Autodesk Fusion 360 part; units mm, degrees
note: some values were not read from the file. Set by a fixed rule: which sketch regions a step uses.
(part 3 of 5)
extrude "Extrude3" cut sketch "Sketch3" against normal blind 0.5 contours L4 L24 L28 L40 L47 L50 L76 L81 L84 L116 L125 L129 L150 L155 L178 L210 L218 L225 L257 L304 L305 L332 L361 L386 L393 L479 L493 L497 L500 L526 L555 L557 L582 L587 L593 L598 L619 L670 L671 L694 L751 L783 L835 L871 L904 L934 L942 L946 L947 L982 L993 L997 L1046 L1064 L1093 L1098 L1104 L1114 L1123 L1124 L1129 L1137 L1150 L1158 L1165 L1171 L1172 L1176 L1181 L1189 L1191 L1213 L1217 L1219 L1221 L1234 L1256 L1262 L1266 L1284 L1287 L1293 L1300 L1301 L1641 L1649 | L5 L15 L17 L21 L38 L41 L43 L49 L59 L61 L88 L107 L123 L132 L157 L161 L208 L221 L227 L247 L256 L262 L264 L279 L300 L345 L359 L366 L367 L390 L394 L395 L403 L405 L423 L433 L494 L502 L515 L531 L534 L535 L548 L553 L576 L595 L655 L672 L678 L724 L733 L787 L806 L822 L852 L853 L861 L864 L870 L920 L961 L970 L976 L989 L995 L1000 L1001 L1004 L1015 L1018 L1027 L1039 L1068 L1069 L1099 L1105 L1140 L1143 L1161 L1168 L1175 L1195 L1196 L1210 L1224 L1240 L1269 L1377 L1625 | L6 L18 L26 L32 L44 L51 L55 L57 L70 L71 L72 L90 L91 L95 L99 L105 L106 L109 L113 L117 L118 L119 L126 L130 L137 L140 L143 L144 L146 L147 L169 L181 L185 L186 L188 L190 L206 L229 L232 L236 L240 L248 L253 L259 L260 L263 L269 L270 L286 L288 L291 L296 L301 L312 L323 L329 L330 L338 L341 L346 L358 L362 L372 L383 L384 L391 L392 L404 L417 L424 L445 L448 L451 L452 L453 L462 L476 L480 L482 L485 L498 L501 L513 L516 L523 L533 L536 L540 L543 L547 L558 L571 L573 L586 L589 L596 L607 L617 L623 L628 L631 L637 L656 L667 L669 L676 L697 L701 L703 L707 L715 L723 L727 L731 L732 L735 L736 L743 L744 L749 L755 L761 L774 L782 L790 L794 L800 L803 L805 L815 L823 L826 L828 L831 L839 L840 L850 L863 L866 L867 L872 L874 L875 L878 L883 L887 L894 L896 L902 L908 L912 L918 L933 L939 L945 L950 L957 L964 L966 L972 L978 L980 L984 L986 L987 L999 L1002 L1008 L1012 L1013 L1016 L1040 L1043 L1044 L1054 L1059 L1062 L1066 L1071 L1072 L1075 L1078 L1079 L1081 L1088 L1094 L1095 L1103 L1106 L1108 L1110 L1111 L1112 L1113 L1131 L1132 L1134 L1141 L1145 L1148 L1159 L1163 L1164 L1169 L1177 L1179 L1185 L1186 L1187 L1207 L1208 L1209 L1211 L1226 L1238 L1243 L1244 L1245 L1246 L1252 L1255 L1264 L1281 L1283 L1294 L1297 L1302 L1331 L1371 L1469 L1482 L1483 L1555 L1574 L1575 L1576 L1580 L1590 L1615 L1616 L1617 L1618 L1619 L1631 L1636 L1644 L1647 L1655 | L7 L8 L14 L25 L31 L33 L48 L100 L111 L134 L151 L164 L173 L183 L191 L197 L198 L200 L201 L209 L216 L223 L233 L246 L252 L258 L265 L278 L281 L282 L314 L324 L327 L335 L336 L339 L348 L364 L369 L382 L387 L388 L389 L407 L408 L411 L414 L415 L426 L435 L438 L441 L442 L446 L449 L456 L457 L458 L469 L470 L475 L477 L478 L484 L488 L492 L496 L504 L507 L510 L511 L512 L517 L519 L521 L524 L529 L532 L539 L542 L545 L546 L549 L550 L552 L559 L562 L567 L575 L577 L578 L580 L583 L592 L597 L600 L606 L608 L612 L613 L616 L618 L620 L624 L626 L629 L632 L633 L635 L639 L640 L641 L642 L643 L644 L646 L647 L649 L650 L653 L658 L659 L660 L661 L662 L663 L665 L668 L673 L674 L679 L681 L683 L684 L685 L686 L690 L691 L692 L693 L695 L696 L700 L702 L705 L710 L713 L726 L737 L739 L756 L758 L759 L763 L764 L765 L770 L780 L781 L785 L789 L791 L793 L795 L799 L801 L811 L813 L817 L821 L837 L842 L845 L847 L848 L851 L855 L857 L858 L859 L860 L877 L890 L891 L936 L937 L1041 L1120 L1147 L1149 L1180 L1183 L1199 L1203 L1206 L1257 L1304 L1306 L1307 L1308 L1309 L1310 L1312 L1313 L1314 L1315 L1317 L1319 L1320 L1321 L1322 L1323 L1325 L1326 L1327 L1328 L1332 L1333 L1334 L1335 L1336 L1337 L1339 L1342 L1367 L1368 L1369 L1372 L1373 L1374 L1375 L1376 L1379 L1380 L1389 L1390 L1391 L1392 L1393 L1394 L1395 L1396 L1398 L1399 L1400 L1401 L1406 L1410 L1411 L1412 L1414 L1415 L1418 L1450 L1452 L1453 L1454 L1455 L1456 L1457 L1458 L1459 L1460 L1461 L1462 L1463 L1464 L1465 L1466 L1467 L1468 | L9 L20 L35 L63 L73 L83 L85 L97 L101 L156 L162 L168 L176 L177 L193 L205 L212 L235 L239 L241 L294 L353 L397 L413 L455 L471 L503 L508 L544 L565 L572 L585 L664 L666 L677 L688 L718 L740 L767 L775 L788 L809 L819 L830 L854 L865 L886 L888 L909 L913 L935 L949 L979 L991 L992 L994 L996 L1038 L1047 L1049 L1067 L1080 L1096 L1117 L1128 L1138 L1142 L1144 L1152 L1153 L1155 L1166 L1174 L1201 L1204 L1205 L1235 L1239 L1241 L1277 L1318 L1620 L1621 L1622 L1623 L1624 L1626 L1627 L1628 L1629 | L10 L13 L58 L66 L75 L78 L79 L86 L98 L120 L142 L196 L204 L234 L261 L298 L373 L385 L422 L454 L474 L486 L528 L591 L615 L675 L680 L689 L719 L762 L818 L820 L825 L829 L879 L884 L885 L893 L907 L916 L928 L967 L983 L990 L1007 L1009 L1017 L1035 L1050 L1063 L1074 L1121 L1139 L1167 L1170 L1173 L1271 L1291 L1630 L1633 L1638 L1639 L1648 L1650 L1651 L1652 | L11 L22 L53 L62 L68 L82 L104 L133 L152 L172 L226 L242 L250 L360 L379 L412 L443 L489 L505 L509 L525 L561 L574 L601 L622 L636 L645 L711 L717 L722 L772 L802 L814 L849 L882 L900 L903 L906 L919 L932 L938 L963 L965 L1051 L1053 L1077 L1109 L1127 L1133 L1136 L1222 L1232 L1237 L1249 L1259 L1289 L1290 L1365 L1428 L1637 L1640 L1646 L1653 L1654 | L12 L19 L27 L29 L30 L36 L37 L42 L45 L46 L52 L54 L56 L60 L67 L69 L74 L77 L80 L87 L89 L93 L94 L102 L110 L112 L114 L115 L124 L131 L135 L136 L138 L141 L153 L159 L160 L167 L171 L175 L180 L192 L199 L202 L217 L220 L224 L228 L230 L231 L244 L245 L251 L266 L283 L287 L290 L297 L299 L303 L307 L309 L315 L321 L322 L328 L331 L333 L334 L349 L352 L354 L365 L368 L370 L376 L396 L398 L399 L402 L427 L450 L460 L465 L468 L472 L483 L487 L490 L491 L495 L514 L520 L522 L527 L537 L541 L551 L554 L560 L563 L566 L568 L570 L579 L584 L602 L604 L611 L651 L657 L682 L698 L704 L706 L708 L709 L720 L741 L747 L748 L750 L760 L768 L769 L773 L778 L808 L816 L824 L827 L832 L834 L846 L862 L868 L869 L876 L881 L889 L895 L910 L911 L914 L926 L927 L929 L944 L948 L951 L962 L971 L977 L981 L985 L988 L998 L1005 L1006 L1010 L1026 L1045 L1055 L1061 L1065 L1070 L1073 L1085 L1091 L1092 L1097 L1118 L1125 L1146 L1151 L1156 L1157 L1160 L1162 L1178 L1182 L1188 L1200 L1220 L1227 L1248 L1251 L1253 L1265 L1274 L1275 L1279 L1286 L1292 L1295 L1296 L1298 L1303 L1370 L1632 L1634 L1635 L1642 L1643 L1645 L1656 | L16 L23 L39 L64 L92 L108 L121 L122 L127 L128 L139 L145 L148 L149 L154 L158 L165 L166 L170 L187 L189 L194 L211 L219 L237 L255 L268 L271 L273 L275 L280 L292 L293 L306 L313 L316 L319 L337 L347 L356 L371 L421 L447 L461 L518 L569 L610 L621 L638 L648 L652 L687 L712 L716 L728 L779 L796 L804 L838 L841 L843 L873 L892 L898 L899 L901 L915 L917 L921 L922 L924 L925 L930 L931 L940 L941 L943 L954 L959 L968 L969 L973 L974 L1003 L1011 L1014 L1019 L1020 L1028 L1029 L1030 L1031 L1032 L1033 L1034 L1036 L1037 L1042 L1048 L1052 L1056 L1057 L1058 L1060 L1076 L1082 L1083 L1084 L1086 L1087 L1089 L1090 L1101 L1107 L1115 L1116 L1122 L1130 L1135 L1154 L1184 L1192 L1193 L1194 L1198 L1202 L1216 L1218 L1225 L1231 L1233 L1236 L1242 L1247 L1250 L1261 L1268 L1270 L1273 L1285 L1299 | L34 L163 L203 L207 L243 L254 L284 L289 L317 L363 L418 L420 L425 L444 L466 L473 L499 L506 L564 L588 L590 L594 L609 L654 L725 L771 L797 L880 L1230 L1278 L1305 L1311 L1316 L1324 L1329 L1330 L1338 L1340 L1341 L1343 L1344 L1345 L1346 L1347 L1348 L1349 L1350 L1351 L1352 L1353 L1354 L1355 L1356 L1357 L1358 L1359 L1360 L1361 L1362 L1363 L1364 L1366 L1378 L1381 L1382 L1383 L1384 L1385 L1386 L1387 L1388 L1397 L1402 L1403 L1404 L1405 L1407 L1408 L1409 L1413 L1416 L1417 L1419 L1420 L1421 L1422 L1423 L1424 L1425 L1426 L1427 L1429 L1430 L1431 L1432 L1433 L1434 L1435 L1436 L1437 L1438 L1439 L1440 L1441 L1442 L1443 L1444 L1445 L1446 L1447 L1448 L1449 L1451 L1470 L1471 L1472 L1473 L1474 L1475 L1476 L1477 L1478 L1479 L1480 L1481 L1484 L1485 L1486 L1487 L1488 L1489 L1490 L1491 L1492 L1493 L1494 L1495 L1496 L1497 L1498 L1499 L1500 L1501 L1502 L1503 L1504 L1505 L1506 L1507 L1508 L1509 L1510 L1511 L1512 L1513 L1514 L1515 L1516 L1517 L1518 L1519 L1520 L1521 L1522 L1523 L1524 L1525 L1526 L1527 L1528 L1529 L1530 L1531 L1532 L1533 L1534 L1535 L1536 L1537 L1538 L1539 L1540 L1541 L1542 L1543 L1544 L1545 L1546 L1547 L1548 L1549 L1550 L1551 L1552 L1553 L1554 L1556 L1557 L1558 L1559 L1560 L1561 L1562 L1563 L1564 L1565 L1566 L1567 L1568 L1569 L1570 L1571 L1572 L1573 L1577 L1578 L1579 L1581 L1582 L1583 L1584 L1585 L1586 L1587 L1588 L1589 L1591 L1592 L1593 L1594 L1595 L1596 L1597 L1598 L1599 L1600 L1601 L1602 L1603 L1604 L1605 L1606 L1607 L1608 L1609 L1610 L1611 L1612 L1613 L1614 | L65 L96 L103 L174 L179 L182 L184 L195 L213 L214 L215 L222 L238 L249 L267 L272 L274 L276 L277 L285 L295 L302 L308 L310 L311 L318 L320 L325 L326 L340 L342 L343 L344 L350 L351 L355 L357 L374 L375 L377 L378 L380 L381 L400 L401 L406 L409 L410 L416 L419 L428 L429 L430 L431 L432 L434 L436 L437 L439 L440 L459 L463 L464 L481 L530 L538 L556 L581 L599 L603 L605 L614 L625 L627 L630 L634 L699 L714 L721 L729 L730 L734 L738 L742 L745 L746 L752 L753 L754 L757 L766 L776 L777 L784 L786 L792 L798 L807 L810 L812 L833 L836 L844 L856 L897 L905 L923 L952 L953 L955 L956 L958 L960 L975 L1021 L1022 L1023 L1024 L1025 L1100 L1102 L1119 L1126 L1190 L1197 L1212 L1214 L1215 L1223 L1228 L1229 L1254 L1258 L1260 L1263 L1267 L1272 L1276 L1280 L1288 in component "PCB Cover"
sketch "DXF" plane through (0, 0, 3) normal (0, 0, 1) x (-1, 0, 0)
  line L0 (-47.0979, -80.9274) -> (-46.9857, -80.9562)
  line L1 (-46.9857, -80.9562) -> (-46.8782, -80.9955)
  line L2 (-46.8782, -80.9955) -> (-46.7759, -81.0448)
  line L3 (-46.7759, -81.0448) -> (-46.6794, -81.1034)
  line L4 (-46.6794, -81.1034) -> (-46.5893, -81.1708)
  line L5 (-46.5893, -81.1708) -> (-46.5062, -81.2463)
  line L6 (-46.5062, -81.2463) -> (-46.4306, -81.3294)
  line L7 (-46.4306, -81.3294) -> (-46.3632, -81.4195)
  line L8 (-46.3632, -81.4195) -> (-46.3046, -81.516)
  line L9 (-46.3046, -81.516) -> (-46.2553, -81.6183)
  line L10 (-46.2553, -81.6183) -> (-46.2159, -81.7259)
  line L11 (-46.2159, -81.7259) -> (-46.187, -81.8381)
  line L12 (-46.187, -81.8381) -> (-46.1692, -81.9544)
  line L13 (-46.1692, -81.9544) -> (-46.1632, -82.0741)
  line L14 (-46.1632, -82.0741) -> (-46.1692, -82.1938)
  line L15 (-46.1692, -82.1938) -> (-46.187, -82.31)
  line L16 (-46.187, -82.31) -> (-46.2159, -82.4222)
  line L17 (-46.2159, -82.4222) -> (-46.2553, -82.5297)
  line L18 (-46.2553, -82.5297) -> (-46.3046, -82.632)
  line L19 (-46.3046, -82.632) -> (-46.3632, -82.7285)
  line L20 (-46.3632, -82.7285) -> (-46.4306, -82.8186)
  line L21 (-46.4306, -82.8186) -> (-46.5062, -82.9017)
  line L22 (-46.5062, -82.9017) -> (-46.5893, -82.9773)
  line L23 (-46.5893, -82.9773) -> (-46.6794, -83.0447)
  line L24 (-46.6794, -83.0447) -> (-46.7759, -83.1033)
  line L25 (-46.7759, -83.1033) -> (-46.8782, -83.1526)
  line L26 (-46.8782, -83.1526) -> (-46.9857, -83.192)
  line L27 (-46.9857, -83.192) -> (-47.0979, -83.2208)
  line L28 (-47.0979, -83.2208) -> (-47.2141, -83.2385)
  line L29 (-47.2141, -83.2385) -> (-47.3337, -83.2445)
  line L30 (-47.3337, -83.2445) -> (-52.2486, -83.2445)
  line L31 (-52.2486, -83.2445) -> (-52.3978, -83.2329)
  line L32 (-52.3978, -83.2329) -> (-52.5415, -83.2028)
  line L33 (-52.5415, -83.2028) -> (-52.7317, -83.1755)
  line L34 (-52.7317, -83.1755) -> (-52.9126, -83.1337)
  line L35 (-52.9126, -83.1337) -> (-53.0837, -83.0778)
  line L36 (-53.0837, -83.0778) -> (-53.2446, -83.0083)
  line L37 (-53.2446, -83.0083) -> (-53.395, -82.9256)
  line L38 (-53.395, -82.9256) -> (-53.5344, -82.8302)
  line L39 (-53.5344, -82.8302) -> (-53.6624, -82.7225)
  line L40 (-53.6624, -82.7225) -> (-53.7786, -82.603)
  line L41 (-53.7786, -82.603) -> (-53.8827, -82.4721)
  line L42 (-53.8827, -82.4721) -> (-53.9742, -82.3302)
  line L43 (-53.9742, -82.3302) -> (-54.0527, -82.1779)
  line L44 (-54.0527, -82.1779) -> (-54.1178, -82.0155)
  line L45 (-54.1178, -82.0155) -> (-54.1692, -81.8436)
  line L46 (-54.1692, -81.8436) -> (-54.2064, -81.6625)
  line L47 (-54.2064, -81.6625) -> (-54.229, -81.4727)
  line L48 (-54.229, -81.4727) -> (-54.237, -81.2746)
  line L49 (-54.237, -81.2746) -> (-54.237, -71.9056)
  line L50 (-54.237, -71.9056) -> (-54.241, -71.6908)
  line L51 (-54.241, -71.6908) -> (-54.2524, -71.4835)
  line L52 (-54.2524, -71.4835) -> (-54.2713, -71.2837)
  line L53 (-54.2713, -71.2837) -> (-54.2977, -71.0913)
  line L54 (-54.2977, -71.0913) -> (-54.3315, -70.9062)
  line L55 (-54.3315, -70.9062) -> (-54.3726, -70.7284)
  line L56 (-54.3726, -70.7284) -> (-54.4209, -70.5579)
  line L57 (-54.4209, -70.5579) -> (-54.4764, -70.3947)
  line L58 (-54.4764, -70.3947) -> (-54.539, -70.2386)
  line L59 (-54.539, -70.2386) -> (-54.6086, -70.0896)
  line L60 (-54.6086, -70.0896) -> (-54.6852, -69.9478)
  line L61 (-54.6852, -69.9478) -> (-54.7687, -69.813)
  line L62 (-54.7687, -69.813) -> (-54.859, -69.6851)
  line L63 (-54.859, -69.6851) -> (-54.9561, -69.5643)
  line L64 (-54.9561, -69.5643) -> (-55.0598, -69.4503)
  line L65 (-55.0598, -69.4503) -> (-55.1702, -69.3433)
  line L66 (-55.1702, -69.3433) -> (-55.2872, -69.243)
  line L67 (-55.2872, -69.243) -> (-55.4106, -69.1495)
  line L68 (-55.4106, -69.1495) -> (-55.5404, -69.0628)
  line L69 (-55.5404, -69.0628) -> (-55.6766, -68.9828)
  line L70 (-55.6766, -68.9828) -> (-55.8191, -68.9094)
  line L71 (-55.8191, -68.9094) -> (-55.9677, -68.8427)
  line L72 (-55.9677, -68.8427) -> (-56.1225, -68.7825)
  line L73 (-56.1225, -68.7825) -> (-56.2833, -68.7288)
  line L74 (-56.2833, -68.7288) -> (-56.4502, -68.6816)
  line L75 (-56.4502, -68.6816) -> (-56.6229, -68.6408)
  line L76 (-56.6229, -68.6408) -> (-56.986, -68.5784)
  line L77 (-56.986, -68.5784) -> (-57.3718, -68.5413)
  line L78 (-57.3718, -68.5413) -> (-57.78, -68.5289)
  line L79 (-57.78, -68.5289) -> (-58.1882, -68.5413)
  line L80 (-58.1882, -68.5413) -> (-58.574, -68.5784)
  line L81 (-58.574, -68.5784) -> (-58.937, -68.6408)
  line L82 (-58.937, -68.6408) -> (-59.1098, -68.6816)
  line L83 (-59.1098, -68.6816) -> (-59.2767, -68.7288)
  line L84 (-59.2767, -68.7288) -> (-59.4375, -68.7825)
  line L85 (-59.4375, -68.7825) -> (-59.5923, -68.8427)
  line L86 (-59.5923, -68.8427) -> (-59.741, -68.9094)
  line L87 (-59.741, -68.9094) -> (-59.8834, -68.9828)
  line L88 (-59.8834, -68.9828) -> (-60.0196, -69.0628)
  line L89 (-60.0196, -69.0628) -> (-60.1495, -69.1495)
  line L90 (-60.1495, -69.1495) -> (-60.2729, -69.243)
  line L91 (-60.2729, -69.243) -> (-60.3899, -69.3433)
  line L92 (-60.3899, -69.3433) -> (-60.5003, -69.4503)
  line L93 (-60.5003, -69.4503) -> (-60.6041, -69.5643)
  line L94 (-60.6041, -69.5643) -> (-60.7012, -69.6851)
  line L95 (-60.7012, -69.6851) -> (-60.7916, -69.813)
  line L96 (-60.7916, -69.813) -> (-60.8751, -69.9478)
  line L97 (-60.8751, -69.9478) -> (-60.9517, -70.0896)
  line L98 (-60.9517, -70.0896) -> (-61.0214, -70.2386)
  line L99 (-61.0214, -70.2386) -> (-61.084, -70.3947)
  line L100 (-61.084, -70.3947) -> (-61.1395, -70.5579)
  line L101 (-61.1395, -70.5579) -> (-61.1878, -70.7284)
  line L102 (-61.1878, -70.7284) -> (-61.2289, -70.9062)
  line L103 (-61.2289, -70.9062) -> (-61.2627, -71.0913)
  line L104 (-61.2627, -71.0913) -> (-61.2891, -71.2837)
  line L105 (-61.2891, -71.2837) -> (-61.3081, -71.4835)
  line L106 (-61.3081, -71.4835) -> (-61.3195, -71.6908)
  line L107 (-61.3195, -71.6908) -> (-61.3235, -71.9056)
  line L108 (-61.3235, -71.9056) -> (-61.3235, -81.2746)
  line L109 (-61.3235, -81.2746) -> (-61.3325, -81.4884)
  line L110 (-61.3325, -81.4884) -> (-61.3587, -81.6928)
  line L111 (-61.3587, -81.6928) -> (-61.4018, -81.887)
  line L112 (-61.4018, -81.887) -> (-61.4612, -82.0706)
  line L113 (-61.4612, -82.0706) -> (-61.5365, -82.243)
  line L114 (-61.5365, -82.243) -> (-61.6272, -82.4034)
  line L115 (-61.6272, -82.4034) -> (-61.7328, -82.5514)
  line L116 (-61.7328, -82.5514) -> (-61.8529, -82.6864)
  line L117 (-61.8529, -82.6864) -> (-61.9869, -82.8077)
  line L118 (-61.9869, -82.8077) -> (-62.1343, -82.9148)
  line L119 (-62.1343, -82.9148) -> (-62.2947, -83.007)
  line L120 (-62.2947, -83.007) -> (-62.4675, -83.0838)
  line L121 (-62.4675, -83.0838) -> (-62.6523, -83.1446)
  line L122 (-62.6523, -83.1446) -> (-62.8487, -83.1888)
  line L123 (-62.8487, -83.1888) -> (-63.056, -83.2157)
  line L124 (-63.056, -83.2157) -> (-63.2738, -83.2247)
  line L125 (-63.2738, -83.2247) -> (-63.4915, -83.2157)
  line L126 (-63.4915, -83.2157) -> (-63.6988, -83.1888)
  line L127 (-63.6988, -83.1888) -> (-63.895, -83.1446)
  line L128 (-63.895, -83.1446) -> (-64.0798, -83.0838)
  line L129 (-64.0798, -83.0838) -> (-64.2526, -83.007)
  line L130 (-64.2526, -83.007) -> (-64.4129, -82.9148)
  line L131 (-64.4129, -82.9148) -> (-64.5603, -82.8077)
  line L132 (-64.5603, -82.8077) -> (-64.6942, -82.6864)
  line L133 (-64.6942, -82.6864) -> (-64.8142, -82.5514)
  line L134 (-64.8142, -82.5514) -> (-64.9198, -82.4034)
  line L135 (-64.9198, -82.4034) -> (-65.0105, -82.243)
  line L136 (-65.0105, -82.243) -> (-65.0858, -82.0706)
  line L137 (-65.0858, -82.0706) -> (-65.1452, -81.887)
  line L138 (-65.1452, -81.887) -> (-65.1882, -81.6928)
  line L139 (-65.1882, -81.6928) -> (-65.2144, -81.4884)
  line L140 (-65.2144, -81.4884) -> (-65.2234, -81.2746)
  line L141 (-65.2234, -81.2746) -> (-65.2234, -72.2146)
  line L142 (-65.2234, -72.2146) -> (-65.2174, -72.0012)
  line L143 (-65.2174, -72.0012) -> (-65.207, -71.7916)
  line L144 (-65.207, -71.7916) -> (-65.2215, -71.648)
  line L145 (-65.2215, -71.648) -> (-65.2235, -67.8035)
  line L146 (-65.2235, -67.8035) -> (-65.3418, -67.7972)
  line L147 (-65.3418, -67.7972) -> (-65.458, -67.7795)
  line L148 (-65.458, -67.7795) -> (-65.5702, -67.7507)
  line L149 (-65.5702, -67.7507) -> (-65.6778, -67.7114)
  line L150 (-65.6778, -67.7114) -> (-65.7801, -67.6622)
  line L151 (-65.7801, -67.6622) -> (-65.8766, -67.6036)
  line L152 (-65.8766, -67.6036) -> (-65.9667, -67.5363)
  line L153 (-65.9667, -67.5363) -> (-66.0499, -67.4608)
  line L154 (-66.0499, -67.4608) -> (-66.1255, -67.3777)
  line L155 (-66.1255, -67.3777) -> (-66.1929, -67.2877)
  line L156 (-66.1929, -67.2877) -> (-66.2516, -67.1913)
  line L157 (-66.2516, -67.1913) -> (-66.3009, -67.089)
  line L158 (-66.3009, -67.089) -> (-66.3403, -66.9815)
  line L159 (-66.3403, -66.9815) -> (-66.3691, -66.8694)
  line L160 (-66.3691, -66.8694) -> (-66.3868, -66.7532)
  line L161 (-66.3868, -66.7532) -> (-66.3928, -66.6336)
  line L162 (-66.3928, -66.6336) -> (-66.3868, -66.514)
  line L163 (-66.3868, -66.514) -> (-66.3691, -66.3979)
  line L164 (-66.3691, -66.3979) -> (-66.3403, -66.2857)
  line L165 (-66.3403, -66.2857) -> (-66.3009, -66.1782)
  line L166 (-66.3009, -66.1782) -> (-66.2516, -66.076)
  line L167 (-66.2516, -66.076) -> (-66.1929, -65.9795)
  line L168 (-66.1929, -65.9795) -> (-66.1255, -65.8894)
  line L169 (-66.1255, -65.8894) -> (-66.0499, -65.8063)
  line L170 (-66.0499, -65.8063) -> (-65.9667, -65.7308)
  line L171 (-65.9667, -65.7308) -> (-65.8766, -65.6634)
  line L172 (-65.8766, -65.6634) -> (-65.7801, -65.6048)
  line L173 (-65.7801, -65.6048) -> (-65.6778, -65.5555)
  line L174 (-65.6778, -65.5555) -> (-65.5702, -65.5161)
  line L175 (-65.5702, -65.5161) -> (-65.458, -65.4873)
  line L176 (-65.458, -65.4873) -> (-65.3418, -65.4696)
  line L177 (-65.3418, -65.4696) -> (-65.222, -65.4636)
  line L178 (-65.222, -65.4636) -> (-64.0494, -65.4636)
  line L179 (-64.0494, -65.4636) -> (-63.9298, -65.4696)
  line L180 (-63.9298, -65.4696) -> (-63.8136, -65.4873)
  line L181 (-63.8136, -65.4873) -> (-63.7014, -65.5161)
  line L182 (-63.7014, -65.5161) -> (-63.5939, -65.5555)
  line L183 (-63.5939, -65.5555) -> (-63.4916, -65.6048)
  line L184 (-63.4916, -65.6048) -> (-63.3951, -65.6634)
  line L185 (-63.3951, -65.6634) -> (-63.305, -65.7308)
  line L186 (-63.305, -65.7308) -> (-63.2219, -65.8063)
  line L187 (-63.2219, -65.8063) -> (-63.1464, -65.8894)
  line L188 (-63.1464, -65.8894) -> (-63.079, -65.9795)
  line L189 (-63.079, -65.9795) -> (-63.0204, -66.076)
  line L190 (-63.0204, -66.076) -> (-62.9711, -66.1782)
  line L191 (-62.9711, -66.1782) -> (-62.9317, -66.2857)
  line L192 (-62.9317, -66.2857) -> (-62.9029, -66.3979)
  line L193 (-62.9029, -66.3979) -> (-62.8852, -66.514)
  line L194 (-62.8852, -66.514) -> (-62.8792, -66.6336)
  line L195 (-62.8792, -66.6336) -> (-62.8792, -66.7881)
  line L196 (-62.8792, -66.7881) -> (-62.6352, -66.6169)
  line L197 (-62.6352, -66.6169) -> (-62.3805, -66.4572)
  line L198 (-62.3805, -66.4572) -> (-62.1152, -66.3088)
  line L199 (-62.1152, -66.3088) -> (-61.8395, -66.1717)
  line L200 (-61.8395, -66.1717) -> (-61.5536, -66.0458)
  line L201 (-61.5536, -66.0458) -> (-61.2576, -65.9312)
  line L202 (-61.2576, -65.9312) -> (-60.9517, -65.8277)
  line L203 (-60.9517, -65.8277) -> (-60.6361, -65.7353)
  line L204 (-60.6361, -65.7353) -> (-60.3108, -65.654)
  line L205 (-60.3108, -65.654) -> (-59.9762, -65.5837)
  line L206 (-59.9762, -65.5837) -> (-59.6322, -65.5243)
  line L207 (-59.6322, -65.5243) -> (-59.2792, -65.4759)
  line L208 (-59.2792, -65.4759) -> (-58.9172, -65.4383)
  line L209 (-58.9172, -65.4383) -> (-58.5464, -65.4115)
  line L210 (-58.5464, -65.4115) -> (-58.167, -65.3954)
  line L211 (-58.167, -65.3954) -> (-57.7791, -65.3904)
  line L212 (-57.7791, -65.3904) -> (-57.3582, -65.3964)
  line L213 (-57.3582, -65.3964) -> (-56.9471, -65.4152)
  line L214 (-56.9471, -65.4152) -> (-56.5461, -65.4465)
  line L215 (-56.5461, -65.4465) -> (-56.1554, -65.4904)
  line L216 (-56.1554, -65.4904) -> (-55.7752, -65.5471)
  line L217 (-55.7752, -65.5471) -> (-55.4058, -65.6166)
  line L218 (-55.4058, -65.6166) -> (-55.0473, -65.699)
  line L219 (-55.0473, -65.699) -> (-54.7002, -65.7945)
  line L220 (-54.7002, -65.7945) -> (-54.3644, -65.9031)
  line L221 (-54.3644, -65.9031) -> (-54.0404, -66.0248)
  line L222 (-54.0404, -66.0248) -> (-53.7283, -66.1599)
  line L223 (-53.7283, -66.1599) -> (-53.4283, -66.3082)
  line L224 (-53.4283, -66.3082) -> (-53.1407, -66.4701)
  line L225 (-53.1407, -66.4701) -> (-52.8657, -66.6454)
  line L226 (-52.8657, -66.6454) -> (-52.6036, -66.8344)
  line L227 (-52.6036, -66.8344) -> (-52.3545, -67.0371)
  line L228 (-52.3545, -67.0371) -> (-52.1188, -67.2535)
  line L229 (-52.1188, -67.2535) -> (-51.8966, -67.4839)
  line L230 (-51.8966, -67.4839) -> (-51.6881, -67.7282)
  line L231 (-51.6881, -67.7282) -> (-51.4937, -67.9865)
  line L232 (-51.4937, -67.9865) -> (-51.3135, -68.2591)
  line L233 (-51.3135, -68.2591) -> (-51.1477, -68.5458)
  line L234 (-51.1477, -68.5458) -> (-50.9966, -68.8468)
  line L235 (-50.9966, -68.8468) -> (-50.8605, -69.1623)
  line L236 (-50.8605, -69.1623) -> (-50.7395, -69.4922)
  line L237 (-50.7395, -69.4922) -> (-50.6339, -69.8368)
  line L238 (-50.6339, -69.8368) -> (-50.5439, -70.1959)
  line L239 (-50.5439, -70.1959) -> (-50.4697, -70.5698)
  line L240 (-50.4697, -70.5698) -> (-50.4116, -70.9586)
  line L241 (-50.4116, -70.9586) -> (-50.3698, -71.3623)
  line L242 (-50.3698, -71.3623) -> (-50.3446, -71.781)
  line L243 (-50.3446, -71.781) -> (-50.3366, -72.2147)
  line L244 (-50.3366, -72.2147) -> (-50.3366, -80.9037)
  line L245 (-50.3366, -80.9037) -> (-47.3337, -80.9037)
  line L246 (-47.3337, -80.9037) -> (-47.2141, -80.9097)
  line L247 (-47.2141, -80.9097) -> (-47.0979, -80.9274)
  line L248 (-134.2971, -82.2404) -> (-134.3507, -82.0716)
  line L249 (-134.3507, -82.0716) -> (-134.3896, -81.8899)
  line L250 (-134.3896, -81.8899) -> (-134.4133, -81.6953)
  line L251 (-134.4133, -81.6953) -> (-134.4213, -81.4877)
  line L252 (-134.4213, -81.4877) -> (-134.4213, -67.22)
  line L253 (-134.4213, -67.22) -> (-134.4133, -67.0124)
  line L254 (-134.4133, -67.0124) -> (-134.3896, -66.8178)
  line L255 (-134.3896, -66.8178) -> (-134.3507, -66.6361)
  line L256 (-134.3507, -66.6361) -> (-134.2971, -66.4674)
  line L257 (-134.2971, -66.4674) -> (-134.2293, -66.3118)
  line L258 (-134.2293, -66.3118) -> (-134.1478, -66.1694)
  line L259 (-134.1478, -66.1694) -> (-134.053, -66.0402)
  line L260 (-134.053, -66.0402) -> (-133.9455, -65.9244)
  line L261 (-133.9455, -65.9244) -> (-133.8257, -65.8219)
  line L262 (-133.8257, -65.8219) -> (-133.6942, -65.7328)
  line L263 (-133.6942, -65.7328) -> (-133.5514, -65.6573)
  line L264 (-133.5514, -65.6573) -> (-133.3978, -65.5954)
  line L265 (-133.3978, -65.5954) -> (-133.2339, -65.5471)
  line L266 (-133.2339, -65.5471) -> (-133.0602, -65.5125)
  line L267 (-133.0602, -65.5125) -> (-132.8771, -65.4916)
  line L268 (-132.8771, -65.4916) -> (-132.6853, -65.4846)
  line L269 (-132.6853, -65.4846) -> (-132.4933, -65.4916)
  line L270 (-132.4933, -65.4916) -> (-132.3103, -65.5125)
  line L271 (-132.3103, -65.5125) -> (-132.1365, -65.5471)
  line L272 (-132.1365, -65.5471) -> (-131.9726, -65.5954)
  line L273 (-131.9726, -65.5954) -> (-131.819, -65.6573)
  line L274 (-131.819, -65.6573) -> (-131.6763, -65.7328)
  line L275 (-131.6763, -65.7328) -> (-131.5448, -65.8219)
  line L276 (-131.5448, -65.8219) -> (-131.425, -65.9244)
  line L277 (-131.425, -65.9244) -> (-131.3176, -66.0402)
  line L278 (-131.3176, -66.0402) -> (-131.2229, -66.1694)
  line L279 (-131.2229, -66.1694) -> (-131.1414, -66.3118)
  line L280 (-131.1414, -66.3118) -> (-131.0736, -66.4674)
  line L281 (-131.0736, -66.4674) -> (-131.0201, -66.6361)
  line L282 (-131.0201, -66.6361) -> (-130.9813, -66.8178)
  line L283 (-130.9813, -66.8178) -> (-130.9576, -67.0124)
  line L284 (-130.9576, -67.0124) -> (-130.9496, -67.22)
  line L285 (-130.9496, -67.22) -> (-130.9496, -80.9028)
  line L286 (-130.9496, -80.9028) -> (-130.5171, -80.9028)
  line L287 (-130.5171, -80.9028) -> (-130.3974, -80.9088)
  line L288 (-130.3974, -80.9088) -> (-130.2812, -80.9265)
  line L289 (-130.2812, -80.9265) -> (-130.1691, -80.9553)
  line L290 (-130.1691, -80.9553) -> (-130.0616, -80.9946)
  line L291 (-130.0616, -80.9946) -> (-129.9593, -81.0439)
  line L292 (-129.9593, -81.0439) -> (-129.8628, -81.1025)
  line L293 (-129.8628, -81.1025) -> (-129.7727, -81.1699)
  line L294 (-129.7727, -81.1699) -> (-129.6896, -81.2454)
  line L295 (-129.6896, -81.2454) -> (-129.6141, -81.3285)
  line L296 (-129.6141, -81.3285) -> (-129.5467, -81.4186)
  line L297 (-129.5467, -81.4186) -> (-129.4881, -81.5151)
  line L298 (-129.4881, -81.5151) -> (-129.4388, -81.6175)
  line L299 (-129.4388, -81.6175) -> (-129.3995, -81.725)
  line L300 (-129.3995, -81.725) -> (-129.3707, -81.8373)
  line L301 (-129.3707, -81.8373) -> (-129.353, -81.9536)
  line L302 (-129.353, -81.9536) -> (-129.347, -82.0733)
  line L303 (-129.347, -82.0733) -> (-129.353, -82.193)
  line L304 (-129.353, -82.193) -> (-129.3707, -82.3092)
  line L305 (-129.3707, -82.3092) -> (-129.3995, -82.4213)
  line L306 (-129.3995, -82.4213) -> (-129.4388, -82.5289)
  line L307 (-129.4388, -82.5289) -> (-129.4881, -82.6312)
  line L308 (-129.4881, -82.6312) -> (-129.5467, -82.7277)
  line L309 (-129.5467, -82.7277) -> (-129.6141, -82.8178)
  line L310 (-129.6141, -82.8178) -> (-129.6896, -82.9009)
  line L311 (-129.6896, -82.9009) -> (-129.7727, -82.9765)
  line L312 (-129.7727, -82.9765) -> (-129.8628, -83.0439)
  line L313 (-129.8628, -83.0439) -> (-129.9593, -83.1025)
  line L314 (-129.9593, -83.1025) -> (-130.0616, -83.1518)
  line L315 (-130.0616, -83.1518) -> (-130.1691, -83.1912)
  line L316 (-130.1691, -83.1912) -> (-130.2812, -83.22)
  line L317 (-130.2812, -83.22) -> (-130.3974, -83.2377)
  line L318 (-130.3974, -83.2377) -> (-130.5171, -83.2437)
  line L319 (-130.5171, -83.2437) -> (-132.3759, -83.2437)
  line L320 (-132.3759, -83.2437) -> (-132.4975, -83.2377)
  line L321 (-132.4975, -83.2377) -> (-132.6154, -83.2188)
  line L322 (-132.6154, -83.2188) -> (-132.6852, -83.2248)
  line L323 (-132.6852, -83.2248) -> (-132.8771, -83.2173)
  line L324 (-132.8771, -83.2173) -> (-133.0602, -83.1964)
  line L325 (-133.0602, -83.1964) -> (-133.2339, -83.1617)
  line L326 (-133.2339, -83.1617) -> (-133.3978, -83.1133)
  line L327 (-133.3978, -83.1133) -> (-133.5514, -83.0512)
  line L328 (-133.5514, -83.0512) -> (-133.6942, -82.9756)
  line L329 (-133.6942, -82.9756) -> (-133.8257, -82.8864)
  line L330 (-133.8257, -82.8864) -> (-133.9455, -82.7838)
  line L331 (-133.9455, -82.7838) -> (-134.053, -82.6678)
  line L332 (-134.053, -82.6678) -> (-134.1478, -82.5385)
  line L333 (-134.1478, -82.5385) -> (-134.2293, -82.396)
  line L334 (-134.2293, -82.396) -> (-134.2971, -82.2404)
  line L335 (-141.9397, -65.6991) -> (-141.7958, -65.6248)
  line L336 (-141.7958, -65.6248) -> (-141.644, -65.5652)
  line L337 (-141.644, -65.5652) -> (-141.485, -65.5212)
  line L338 (-141.485, -65.5212) -> (-141.3194, -65.4941)
  line L339 (-141.3194, -65.4941) -> (-141.1482, -65.4851)
  line L340 (-141.1482, -65.4851) -> (-140.9924, -65.4901)
  line L341 (-140.9924, -65.4901) -> (-140.8458, -65.5044)
  line L342 (-140.8458, -65.5044) -> (-140.708, -65.5271)
  line L343 (-140.708, -65.5271) -> (-140.5788, -65.5579)
  line L344 (-140.5788, -65.5579) -> (-140.4577, -65.5959)
  line L345 (-140.4577, -65.5959) -> (-140.3446, -65.6405)
  line L346 (-140.3446, -65.6405) -> (-140.2391, -65.691)
  line L347 (-140.2391, -65.691) -> (-140.1409, -65.7466)
  line L348 (-140.1409, -65.7466) -> (-139.965, -65.8704)
  line L349 (-139.965, -65.8704) -> (-139.8145, -66.0066)
  line L350 (-139.8145, -66.0066) -> (-139.6868, -66.1494)
  line L351 (-139.6868, -66.1494) -> (-139.5794, -66.2933)
  line L352 (-139.5794, -66.2933) -> (-136.2972, -70.9305)
  line L353 (-136.2972, -70.9305) -> (-136.1478, -71.1145)
  line L354 (-136.1478, -71.1145) -> (-135.9986, -71.3165)
  line L355 (-135.9986, -71.3165) -> (-135.8284, -71.5777)
  line L356 (-135.8284, -71.5777) -> (-135.6585, -71.8872)
  line L357 (-135.6585, -71.8872) -> (-135.5805, -72.0567)
  line L358 (-135.5805, -72.0567) -> (-135.5106, -72.2342)
  line L359 (-135.5106, -72.2342) -> (-135.4516, -72.4184)
  line L360 (-135.4516, -72.4184) -> (-135.4061, -72.608)
  line L361 (-135.4061, -72.608) -> (-135.3769, -72.8016)
  line L362 (-135.3769, -72.8016) -> (-135.3666, -72.9978)
  line L363 (-135.3666, -72.9978) -> (-135.3726, -73.1817)
  line L364 (-135.3726, -73.1817) -> (-135.39, -73.3534)
  line L365 (-135.39, -73.3534) -> (-135.417, -73.5132)
  line L366 (-135.417, -73.5132) -> (-135.4521, -73.6609)
  line L367 (-135.4521, -73.6609) -> (-135.4936, -73.7968)
  line L368 (-135.4936, -73.7968) -> (-135.54, -73.9208)
  line L369 (-135.54, -73.9208) -> (-135.641, -74.1334)
  line L370 (-135.641, -74.1334) -> (-135.7422, -74.2993)
  line L371 (-135.7422, -74.2993) -> (-135.8309, -74.4188)
  line L372 (-135.8309, -74.4188) -> (-135.9197, -74.5208)
  line L373 (-135.9197, -74.5208) -> (-138.937, -77.8736)
  line L374 (-138.937, -77.8736) -> (-139.075, -78.0114)
  line L375 (-139.075, -78.0114) -> (-139.2218, -78.1381)
  line L376 (-139.2218, -78.1381) -> (-139.3769, -78.2514)
  line L377 (-139.3769, -78.2514) -> (-139.5402, -78.3492)
  line L378 (-139.5402, -78.3492) -> (-139.7112, -78.4291)
  line L379 (-139.7112, -78.4291) -> (-139.8899, -78.489)
  line L380 (-139.8899, -78.489) -> (-140.0758, -78.5266)
  line L381 (-140.0758, -78.5266) -> (-140.2687, -78.5396)
  line L382 (-140.2687, -78.5396) -> (-140.4165, -78.5316)
  line L383 (-140.4165, -78.5316) -> (-140.5646, -78.5082)
  line L384 (-140.5646, -78.5082) -> (-140.7116, -78.4701)
  line L385 (-140.7116, -78.4701) -> (-140.8562, -78.4181)
  line L386 (-140.8562, -78.4181) -> (-140.997, -78.3528)
  line L387 (-140.997, -78.3528) -> (-141.1327, -78.275)
  line L388 (-141.1327, -78.275) -> (-141.2619, -78.1855)
  line L389 (-141.2619, -78.1855) -> (-141.3833, -78.0849)
  line L390 (-141.3833, -78.0849) -> (-141.4955, -77.9741)
  line L391 (-141.4955, -77.9741) -> (-141.5971, -77.8536)
  line L392 (-141.5971, -77.8536) -> (-141.6868, -77.7243)
  line L393 (-141.6868, -77.7243) -> (-141.7632, -77.5869)
  line L394 (-141.7632, -77.5869) -> (-141.825, -77.4421)
  line L395 (-141.825, -77.4421) -> (-141.8708, -77.2907)
  line L396 (-141.8708, -77.2907) -> (-141.8993, -77.1333)
  line L397 (-141.8993, -77.1333) -> (-141.9093, -76.9708)
  line L398 (-141.9093, -76.9708) -> (-141.8993, -76.7576)
  line L399 (-141.8993, -76.7576) -> (-141.8708, -76.5779)
  line L400 (-141.8708, -76.5779) -> (-141.8251, -76.4251)
  line L401 (-141.8251, -76.4251) -> (-141.7635, -76.2923)
  line L402 (-141.7635, -76.2923) -> (-141.6874, -76.173)
  line L403 (-141.6874, -76.173) -> (-141.5982, -76.0604)
  line L404 (-141.5982, -76.0604) -> (-141.3861, -75.8284)
  line L405 (-141.3861, -75.8284) -> (-138.8179, -73.1413)
  line L406 (-138.8179, -73.1413) -> (-142.4321, -68.291)
  line L407 (-142.4321, -68.291) -> (-142.5381, -68.1262)
  line L408 (-142.5381, -68.1262) -> (-142.5973, -68.0144)
  line L409 (-142.5973, -68.0144) -> (-142.6551, -67.8835)
  line L410 (-142.6551, -67.8835) -> (-142.7073, -67.7335)
  line L411 (-142.7073, -67.7335) -> (-142.7498, -67.5649)
  line L412 (-142.7498, -67.5649) -> (-142.7784, -67.3778)
  line L413 (-142.7784, -67.3778) -> (-142.7888, -67.1725)
  line L414 (-142.7888, -67.1725) -> (-142.7808, -67.0086)
  line L415 (-142.7808, -67.0086) -> (-142.7566, -66.8474)
  line L416 (-142.7566, -66.8474) -> (-142.7171, -66.6901)
  line L417 (-142.7171, -66.6901) -> (-142.6631, -66.5377)
  line L418 (-142.6631, -66.5377) -> (-142.5953, -66.3913)
  line L419 (-142.5953, -66.3913) -> (-142.5144, -66.252)
  line L420 (-142.5144, -66.252) -> (-142.4212, -66.1208)
  line L421 (-142.4212, -66.1208) -> (-142.3164, -65.9988)
  line L422 (-142.3164, -65.9988) -> (-142.2007, -65.8871)
  line L423 (-142.2007, -65.8871) -> (-142.0749, -65.7869)
  line L424 (-142.0749, -65.7869) -> (-141.9397, -65.6991)
  line L425 (-166.0715, -78.5875) -> (-166.2167, -78.5935)
  line L426 (-166.2167, -78.5935) -> (-168.1962, -78.5935)
  line L427 (-168.1962, -78.5935) -> (-168.3718, -78.5846)
  line L428 (-168.3718, -78.5846) -> (-168.5423, -78.5586)
  line L429 (-168.5423, -78.5586) -> (-168.7068, -78.5163)
  line L430 (-168.7068, -78.5163) -> (-168.8644, -78.4586)
  line L431 (-168.8644, -78.4586) -> (-169.0144, -78.3864)
  line L432 (-169.0144, -78.3864) -> (-169.1558, -78.3005)
  line L433 (-169.1558, -78.3005) -> (-169.2879, -78.2018)
  line L434 (-169.2879, -78.2018) -> (-169.4097, -78.0911)
  line L435 (-169.4097, -78.0911) -> (-169.5204, -77.9693)
  line L436 (-169.5204, -77.9693) -> (-169.6191, -77.8372)
  line L437 (-169.6191, -77.8372) -> (-169.705, -77.6958)
  line L438 (-169.705, -77.6958) -> (-169.7772, -77.5459)
  line L439 (-169.7772, -77.5459) -> (-169.8348, -77.3883)
  line L440 (-169.8348, -77.3883) -> (-169.877, -77.2239)
  line L441 (-169.877, -77.2239) -> (-169.903, -77.0537)
  line L442 (-169.903, -77.0537) -> (-169.912, -76.8783)
  line L443 (-169.912, -76.8783) -> (-169.903, -76.7078)
  line L444 (-169.903, -76.7078) -> (-169.877, -76.5517)
  line L445 (-169.877, -76.5517) -> (-169.8348, -76.4096)
  line L446 (-169.8348, -76.4096) -> (-169.7772, -76.2808)
  line L447 (-169.7772, -76.2808) -> (-169.705, -76.165)
  line L448 (-169.705, -76.165) -> (-169.6191, -76.0618)
  line L449 (-169.6191, -76.0618) -> (-169.5204, -75.9706)
  line L450 (-169.5204, -75.9706) -> (-169.4097, -75.8909)
  line L451 (-169.4097, -75.8909) -> (-169.2879, -75.8224)
  line L452 (-169.2879, -75.8224) -> (-169.1558, -75.7645)
  line L453 (-169.1558, -75.7645) -> (-169.0144, -75.7168)
  line L454 (-169.0144, -75.7168) -> (-168.8644, -75.6788)
  line L455 (-168.8644, -75.6788) -> (-168.7068, -75.6501)
  line L456 (-168.7068, -75.6501) -> (-168.5423, -75.63)
  line L457 (-168.5423, -75.63) -> (-168.3718, -75.6183)
  line L458 (-168.3718, -75.6183) -> (-168.1963, -75.6143)
  line L459 (-168.1963, -75.6143) -> (-166.4853, -75.6143)
  line L460 (-166.4853, -75.6143) -> (-164.6445, -74.2229)
  line L461 (-164.6445, -74.2229) -> (-164.6445, -67.2203)
  line L462 (-164.6445, -67.2203) -> (-164.6365, -67.0127)
  line L463 (-164.6365, -67.0127) -> (-164.6128, -66.8181)
  line L464 (-164.6128, -66.8181) -> (-164.5739, -66.6363)
  line L465 (-164.5739, -66.6363) -> (-164.5203, -66.4677)
  line L466 (-164.5203, -66.4677) -> (-164.4525, -66.3121)
  line L467 (-164.4525, -66.3121) -> (-164.3709, -66.1697)
  line L468 (-164.3709, -66.1697) -> (-164.2761, -66.0405)
  line L469 (-164.2761, -66.0405) -> (-164.1686, -65.9247)
  line L470 (-164.1686, -65.9247) -> (-164.0488, -65.8222)
  line L471 (-164.0488, -65.8222) -> (-163.9172, -65.7331)
  line L472 (-163.9172, -65.7331) -> (-163.7744, -65.6576)
  line L473 (-163.7744, -65.6576) -> (-163.6208, -65.5957)
  line L474 (-163.6208, -65.5957) -> (-163.4568, -65.5474)
  line L475 (-163.4568, -65.5474) -> (-163.2831, -65.5128)
  line L476 (-163.2831, -65.5128) -> (-163.1, -65.4919)
  line L477 (-163.1, -65.4919) -> (-162.9082, -65.4849)
  line L478 (-162.9082, -65.4849) -> (-162.7163, -65.4919)
  line L479 (-162.7163, -65.4919) -> (-162.5333, -65.5128)
  line L480 (-162.5333, -65.5128) -> (-162.3596, -65.5474)
  line L481 (-162.3596, -65.5474) -> (-162.1957, -65.5957)
  line L482 (-162.1957, -65.5957) -> (-162.0421, -65.6576)
  line L483 (-162.0421, -65.6576) -> (-161.8993, -65.7331)
  line L484 (-161.8993, -65.7331) -> (-161.7678, -65.8222)
  line L485 (-161.7678, -65.8222) -> (-161.6481, -65.9247)
  line L486 (-161.6481, -65.9247) -> (-161.5406, -66.0405)
  line L487 (-161.5406, -66.0405) -> (-161.4459, -66.1697)
  line L488 (-161.4459, -66.1697) -> (-161.3644, -66.3121)
  line L489 (-161.3644, -66.3121) -> (-161.2966, -66.4677)
  line L490 (-161.2966, -66.4677) -> (-161.243, -66.6363)
  line L491 (-161.243, -66.6363) -> (-161.2041, -66.8181)
  line L492 (-161.2041, -66.8181) -> (-161.1804, -67.0127)
  line L493 (-161.1804, -67.0127) -> (-161.1724, -67.2203)
  line L494 (-161.1724, -67.2203) -> (-161.1724, -76.2193)
  line L495 (-161.1724, -76.2193) -> (-160.7403, -76.2193)
  line L496 (-160.7403, -76.2193) -> (-160.6206, -76.2253)
  line L497 (-160.6206, -76.2253) -> (-160.5044, -76.243)
  line L498 (-160.5044, -76.243) -> (-160.3923, -76.2718)
  line L499 (-160.3923, -76.2718) -> (-160.2848, -76.3111)
  line L500 (-160.2848, -76.3111) -> (-160.1826, -76.3604)
  line L501 (-160.1826, -76.3604) -> (-160.0861, -76.419)
  line L502 (-160.0861, -76.419) -> (-159.996, -76.4863)
  line L503 (-159.996, -76.4863) -> (-159.9129, -76.5618)
  line L504 (-159.9129, -76.5618) -> (-159.8374, -76.6449)
  line L505 (-159.8374, -76.6449) -> (-159.7701, -76.7349)
  line L506 (-159.7701, -76.7349) -> (-159.7115, -76.8314)
  line L507 (-159.7115, -76.8314) -> (-159.6623, -76.9336)
  line L508 (-159.6623, -76.9336) -> (-159.623, -77.0411)
  line L509 (-159.623, -77.0411) -> (-159.5942, -77.1532)
  line L510 (-159.5942, -77.1532) -> (-159.5765, -77.2694)
  line L511 (-159.5765, -77.2694) -> (-159.5705, -77.3891)
  line L512 (-159.5705, -77.3891) -> (-159.5765, -77.5088)
  line L513 (-159.5765, -77.5088) -> (-159.5942, -77.6251)
  line L514 (-159.5942, -77.6251) -> (-159.623, -77.7373)
  line L515 (-159.623, -77.7373) -> (-159.6623, -77.8448)
  line L516 (-159.6623, -77.8448) -> (-159.7115, -77.9471)
  line L517 (-159.7115, -77.9471) -> (-159.7701, -78.0436)
  line L518 (-159.7701, -78.0436) -> (-159.8374, -78.1336)
  line L519 (-159.8374, -78.1336) -> (-159.9129, -78.2166)
  line L520 (-159.9129, -78.2166) -> (-159.996, -78.2921)
  line L521 (-159.996, -78.2921) -> (-160.0861, -78.3594)
  line L522 (-160.0861, -78.3594) -> (-160.1826, -78.4179)
  line L523 (-160.1826, -78.4179) -> (-160.2848, -78.4671)
  line L524 (-160.2848, -78.4671) -> (-160.3923, -78.5064)
  line L525 (-160.3923, -78.5064) -> (-160.5044, -78.5352)
  line L526 (-160.5044, -78.5352) -> (-160.6206, -78.5529)
  line L527 (-160.6206, -78.5529) -> (-160.7403, -78.5589)
  line L528 (-160.7403, -78.5589) -> (-162.5987, -78.5589)
  line L529 (-162.5987, -78.5589) -> (-162.72, -78.5529)
  line L530 (-162.72, -78.5529) -> (-162.8379, -78.5345)
  line L531 (-162.8379, -78.5345) -> (-162.9081, -78.5405)
  line L532 (-162.9081, -78.5405) -> (-163.0667, -78.5355)
  line L533 (-163.0667, -78.5355) -> (-163.2193, -78.5212)
  line L534 (-163.2193, -78.5212) -> (-163.3655, -78.4974)
  line L535 (-163.3655, -78.4974) -> (-163.5051, -78.4641)
  line L536 (-163.5051, -78.4641) -> (-163.6379, -78.4215)
  line L537 (-163.6379, -78.4215) -> (-163.7636, -78.3695)
  line L538 (-163.7636, -78.3695) -> (-163.882, -78.3083)
  line L539 (-163.882, -78.3083) -> (-163.9927, -78.2379)
  line L540 (-163.9927, -78.2379) -> (-164.0956, -78.1584)
  line L541 (-164.0956, -78.1584) -> (-164.1904, -78.0698)
  line L542 (-164.1904, -78.0698) -> (-164.2768, -77.9721)
  line L543 (-164.2768, -77.9721) -> (-164.3546, -77.8655)
  line L544 (-164.3546, -77.8655) -> (-164.4235, -77.7499)
  line L545 (-164.4235, -77.7499) -> (-164.4833, -77.6255)
  line L546 (-164.4833, -77.6255) -> (-164.5337, -77.4924)
  line L547 (-164.5337, -77.4924) -> (-164.5745, -77.3505)
  line L548 (-164.5745, -77.3505) -> (-164.6183, -77.4824)
  line L549 (-164.6183, -77.4824) -> (-164.6721, -77.6095)
  line L550 (-164.6721, -77.6095) -> (-164.7355, -77.7311)
  line L551 (-164.7355, -77.7311) -> (-164.808, -77.8468)
  line L552 (-164.808, -77.8468) -> (-164.8891, -77.9561)
  line L553 (-164.8891, -77.9561) -> (-164.9783, -78.0585)
  line L554 (-164.9783, -78.0585) -> (-165.0752, -78.1535)
  line L555 (-165.0752, -78.1535) -> (-165.1793, -78.2406)
  line L556 (-165.1793, -78.2406) -> (-165.2902, -78.3193)
  line L557 (-165.2902, -78.3193) -> (-165.4074, -78.3891)
  line L558 (-165.4074, -78.3891) -> (-165.5305, -78.4495)
  line L559 (-165.5305, -78.4495) -> (-165.6589, -78.5)
  line L560 (-165.6589, -78.5) -> (-165.7921, -78.5402)
  line L561 (-165.7921, -78.5402) -> (-165.9299, -78.5695)
  line L562 (-165.9299, -78.5695) -> (-166.0715, -78.5875)
  line L563 (-89.4549, -82.9073) -> (-89.5832, -82.7907)
  line L564 (-89.5832, -82.7907) -> (-89.6998, -82.6623)
  line L565 (-89.6998, -82.6623) -> (-89.8038, -82.5231)
  line L566 (-89.8038, -82.5231) -> (-89.8943, -82.3741)
  line L567 (-89.8943, -82.3741) -> (-89.9704, -82.2161)
  line L568 (-89.9704, -82.2161) -> (-90.0311, -82.05)
  line L569 (-90.0311, -82.05) -> (-90.0756, -81.8768)
  line L570 (-90.0756, -81.8768) -> (-90.103, -81.6973)
  line L571 (-90.103, -81.6973) -> (-90.112, -81.5125)
  line L572 (-90.112, -81.5125) -> (-90.103, -81.3276)
  line L573 (-90.103, -81.3276) -> (-90.0756, -81.1482)
  line L574 (-90.0756, -81.1482) -> (-90.0311, -80.975)
  line L575 (-90.0311, -80.975) -> (-89.9704, -80.809)
  line L576 (-89.9704, -80.809) -> (-89.8943, -80.6511)
  line L577 (-89.8943, -80.6511) -> (-89.8038, -80.5021)
  line L578 (-89.8038, -80.5021) -> (-89.6998, -80.3631)
  line L579 (-89.6998, -80.3631) -> (-89.5832, -80.2348)
  line L580 (-89.5832, -80.2348) -> (-89.4549, -80.1182)
  line L581 (-89.4549, -80.1182) -> (-89.3159, -80.0143)
  line L582 (-89.3159, -80.0143) -> (-89.1669, -79.9239)
  line L583 (-89.1669, -79.9239) -> (-89.0089, -79.8479)
  line L584 (-89.0089, -79.8479) -> (-88.8429, -79.7872)
  line L585 (-88.8429, -79.7872) -> (-88.6697, -79.7427)
  line L586 (-88.6697, -79.7427) -> (-88.4902, -79.7153)
  line L587 (-88.4902, -79.7153) -> (-88.3054, -79.7063)
  line L588 (-88.3054, -79.7063) -> (-88.1205, -79.7153)
  line L589 (-88.1205, -79.7153) -> (-87.941, -79.7427)
  line L590 (-87.941, -79.7427) -> (-87.7677, -79.7872)
  line L591 (-87.7677, -79.7872) -> (-87.6017, -79.8479)
  line L592 (-87.6017, -79.8479) -> (-87.4437, -79.9239)
  line L593 (-87.4437, -79.9239) -> (-87.2947, -80.0143)
  line L594 (-87.2947, -80.0143) -> (-87.1556, -80.1182)
  line L595 (-87.1556, -80.1182) -> (-87.0272, -80.2348)
  line L596 (-87.0272, -80.2348) -> (-86.9106, -80.3631)
  line L597 (-86.9106, -80.3631) -> (-86.8066, -80.5021)
  line L598 (-86.8066, -80.5021) -> (-86.7161, -80.6511)
  line L599 (-86.7161, -80.6511) -> (-86.64, -80.809)
  line L600 (-86.64, -80.809) -> (-86.5793, -80.975)
  line L601 (-86.5793, -80.975) -> (-86.5348, -81.1482)
  line L602 (-86.5348, -81.1482) -> (-86.5074, -81.3276)
  line L603 (-86.5074, -81.3276) -> (-86.4984, -81.5125)
  line L604 (-86.4984, -81.5125) -> (-86.5074, -81.6973)
  line L605 (-86.5074, -81.6973) -> (-86.5348, -81.8768)
  line L606 (-86.5348, -81.8768) -> (-86.5793, -82.05)
  line L607 (-86.5793, -82.05) -> (-86.64, -82.2161)
  line L608 (-86.64, -82.2161) -> (-86.7161, -82.3741)
  line L609 (-86.7161, -82.3741) -> (-86.8066, -82.5231)
  line L610 (-86.8066, -82.5231) -> (-86.9106, -82.6623)
  line L611 (-86.9106, -82.6623) -> (-87.0272, -82.7907)
  line L612 (-87.0272, -82.7907) -> (-87.1556, -82.9073)
  line L613 (-87.1556, -82.9073) -> (-87.2947, -83.0114)
  line L614 (-87.2947, -83.0114) -> (-87.4437, -83.1019)
  line L615 (-87.4437, -83.1019) -> (-87.6017, -83.178)
  line L616 (-87.6017, -83.178) -> (-87.7677, -83.2388)
  line L617 (-87.7677, -83.2388) -> (-87.941, -83.2833)
  line L618 (-87.941, -83.2833) -> (-88.1205, -83.3107)
  line L619 (-88.1205, -83.3107) -> (-88.3054, -83.3197)
  line L620 (-88.3054, -83.3197) -> (-88.4902, -83.3107)
  line L621 (-88.4902, -83.3107) -> (-88.6697, -83.2833)
  line L622 (-88.6697, -83.2833) -> (-88.8429, -83.2388)
  line L623 (-88.8429, -83.2388) -> (-89.0089, -83.178)
  line L624 (-89.0089, -83.178) -> (-89.1669, -83.1019)
  line L625 (-89.1669, -83.1019) -> (-89.3159, -83.0114)
  line L626 (-89.3159, -83.0114) -> (-89.4549, -82.9073)
  line L627 (-112.6227, -67.3536) -> (-112.6217, -67.1857)
  line L628 (-112.6217, -67.1857) -> (-112.6041, -67.0202)
  line L629 (-112.6041, -67.0202) -> (-112.5708, -66.858)
  line L630 (-112.5708, -66.858) -> (-112.5222, -66.7004)
  line L631 (-112.5222, -66.7004) -> (-112.459, -66.5484)
  line L632 (-112.459, -66.5484) -> (-112.3816, -66.403)
  line L633 (-112.3816, -66.403) -> (-112.2905, -66.2655)
  line L634 (-112.2905, -66.2655) -> (-112.1863, -66.137)
  line L635 (-112.1863, -66.137) -> (-112.0694, -66.0184)
  line L636 (-112.0694, -66.0184) -> (-111.9405, -65.911)
  line L637 (-111.9405, -65.911) -> (-111.7999, -65.8158)
  line L638 (-111.7999, -65.8158) -> (-111.6483, -65.734)
  line L639 (-111.6483, -65.734) -> (-111.4862, -65.6666)
  line L640 (-111.4862, -65.6666) -> (-111.3423, -65.6222)
  line L641 (-111.3423, -65.6222) -> (-111.1974, -65.591)
  line L642 (-111.1974, -65.591) -> (-111.0523, -65.5725)
  line L643 (-111.0523, -65.5725) -> (-110.908, -65.5665)
  line L644 (-110.908, -65.5665) -> (-110.7765, -65.5715)
  line L645 (-110.7765, -65.5715) -> (-110.6466, -65.5866)
  line L646 (-110.6466, -65.5866) -> (-110.5188, -65.6115)
  line L647 (-110.5188, -65.6115) -> (-110.3937, -65.6458)
  line L648 (-110.3937, -65.6458) -> (-110.2717, -65.6893)
  line L649 (-110.2717, -65.6893) -> (-110.1534, -65.7418)
  line L650 (-110.1534, -65.7418) -> (-110.0394, -65.803)
  line L651 (-110.0394, -65.803) -> (-109.9302, -65.8727)
  line L652 (-109.9302, -65.8727) -> (-109.8263, -65.9506)
  line L653 (-109.8263, -65.9506) -> (-109.7282, -66.0365)
  line L654 (-109.7282, -66.0365) -> (-109.6365, -66.1302)
  line L655 (-109.6365, -66.1302) -> (-109.5517, -66.2313)
  line L656 (-109.5517, -66.2313) -> (-109.4744, -66.3396)
  line L657 (-109.4744, -66.3396) -> (-109.4051, -66.455)
  line L658 (-109.4051, -66.455) -> (-109.3443, -66.577)
  line L659 (-109.3443, -66.577) -> (-109.2926, -66.7055)
  line L660 (-109.2926, -66.7055) -> (-107.0214, -73.0608)
  line L661 (-107.0214, -73.0608) -> (-104.3427, -66.6878)
  line L662 (-104.3427, -66.6878) -> (-104.3357, -66.6717)
  line L663 (-104.3357, -66.6717) -> (-104.2726, -66.5393)
  line L664 (-104.2726, -66.5393) -> (-104.1992, -66.4149)
  line L665 (-104.1992, -66.4149) -> (-104.1537, -66.3521)
  line L666 (-104.1537, -66.3521) -> (-104.086, -66.2611)
  line L667 (-104.086, -66.2611) -> (-104.0125, -66.1757)
  line L668 (-104.0125, -66.1757) -> (-103.9455, -66.1069)
  line L669 (-103.9455, -66.1069) -> (-103.8578, -66.0282)
  line L670 (-103.8578, -66.0282) -> (-103.7659, -65.9563)
  line L671 (-103.7659, -65.9563) -> (-103.7091, -65.9129)
  line L672 (-103.7091, -65.9129) -> (-103.5785, -65.8343)
  line L673 (-103.5785, -65.8343) -> (-103.4417, -65.7676)
  line L674 (-103.4417, -65.7676) -> (-103.4191, -65.7552)
  line L675 (-103.4191, -65.7552) -> (-103.3662, -65.7391)
  line L676 (-103.3662, -65.7391) -> (-103.256, -65.7012)
  line L677 (-103.256, -65.7012) -> (-103.1429, -65.6707)
  line L678 (-103.1429, -65.6707) -> (-103.0505, -65.6498)
  line L679 (-103.0505, -65.6498) -> (-102.906, -65.6294)
  line L680 (-102.906, -65.6294) -> (-102.7591, -65.6214)
  line L681 (-102.7591, -65.6214) -> (-102.7483, -65.6214)
  line L682 (-102.7483, -65.6214) -> (-102.6019, -65.6294)
  line L683 (-102.6019, -65.6294) -> (-102.4573, -65.6498)
  line L684 (-102.4573, -65.6498) -> (-102.3649, -65.6702)
  line L685 (-102.3649, -65.6702) -> (-102.2516, -65.7009)
  line L686 (-102.2516, -65.7009) -> (-102.1409, -65.739)
  line L687 (-102.1409, -65.739) -> (-102.0887, -65.7551)
  line L688 (-102.0887, -65.7551) -> (-102.0665, -65.767)
  line L689 (-102.0665, -65.767) -> (-101.9294, -65.8342)
  line L690 (-101.9294, -65.8342) -> (-101.7987, -65.9127)
  line L691 (-101.7987, -65.9127) -> (-101.743, -65.9554)
  line L692 (-101.743, -65.9554) -> (-101.65, -66.0281)
  line L693 (-101.65, -66.0281) -> (-101.5617, -66.1074)
  line L694 (-101.5617, -66.1074) -> (-101.4961, -66.1748)
  line L695 (-101.4961, -66.1748) -> (-101.4211, -66.2621)
  line L696 (-101.4211, -66.2621) -> (-101.3514, -66.355)
  line L697 (-101.3514, -66.355) -> (-101.3094, -66.4135)
  line L698 (-101.3094, -66.4135) -> (-101.2359, -66.5385)
  line L699 (-101.2359, -66.5385) -> (-101.1722, -66.6714)
  line L700 (-101.1722, -66.6714) -> (-98.4858, -73.0619)
  line L701 (-98.4858, -73.0619) -> (-96.2143, -66.7049)
  line L702 (-96.2143, -66.7049) -> (-96.1626, -66.5764)
  line L703 (-96.1626, -66.5764) -> (-96.1018, -66.4544)
  line L704 (-96.1018, -66.4544) -> (-96.0325, -66.3391)
  line L705 (-96.0325, -66.3391) -> (-95.9551, -66.2307)
  line L706 (-95.9551, -66.2307) -> (-95.8703, -66.1296)
  line L707 (-95.8703, -66.1296) -> (-95.7786, -66.0359)
  line L708 (-95.7786, -66.0359) -> (-95.6805, -65.95)